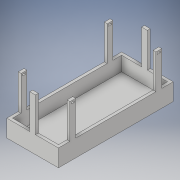
# Autodesk Inventor part: Part1
Saved by Autodesk Inventor 2017 (Build 210142000, 142)
## iProperties
Created: 2017-10-07
Part Number: Part1
Material: Generic
Document SubType Name: Modeling
Designer: User
Density: 1 g/cm^3
Appearance: Default
Author: User
Autodesk Inventor part; units mm, degrees
ref_plane "YZ Plane" through (0, 0, 0) normal (1, 0, 0) x (0, 1, 0)
ref_plane "XZ Plane" through (0, 0, 0) normal (0, 1, 0) x (-1, 0, 0)
ref_plane "XY Plane" through (0, 0, 0) normal (0, 0, 1) x (1, 0, 0)
sketch "Sketch1" plane through (0, 0, 0) normal (0, 1, 0) x (-1, 0, 0)
  line L0 (0, 0) -> (3.175, 0)
  line L1 (3.175, 0) -> (3.175, -3.175)
  line L2 (3.175, -3.175) -> (0, -3.175)
  line L3 (0, -3.175) -> (0, 0)
  line L4 (0, 0) -> (6.35, 0)
  line L5 (0, -6.35) -> (0, 0)
  line L6 (3.175, 0) -> (50.8, 0)
  line L7 (50.8, 0) -> (50.8, -3.175)
  line L8 (50.8, -3.175) -> (3.175, -3.175)
  line L9 (3.175, -3.175) -> (3.175, 0)
  line L10 (50.8, 0) -> (57.15, 0)
  line L11 (57.15, 0) -> (57.15, -6.35)
  line L12 (57.15, 0) -> (53.975, 0)
  line L13 (53.975, 0) -> (53.975, -3.175)
  line L14 (53.975, -3.175) -> (57.15, -3.175)
  line L15 (57.15, -3.175) -> (57.15, 0)
  line L16 (53.975, -120.65) -> (53.975, -123.825)
  line L17 (53.975, -123.825) -> (50.8, -123.825)
  line L18 (57.15, -120.65) -> (57.15, -127)
  line L19 (57.15, -127) -> (50.8, -127)
  line L20 (3.175, -120.65) -> (3.175, -123.825)
  line L21 (3.175, -123.825) -> (6.35, -123.825)
  line L22 (0, -120.65) -> (0, -127)
  line L23 (0, -127) -> (6.35, -127)
  line L24 (53.975, -127) -> (57.15, -127)
  line L25 (57.15, -127) -> (57.15, 0)
  line L26 (57.15, 0) -> (53.975, 0)
  line L27 (53.975, 0) -> (53.975, -127)
  line L28 (50.8, -3.175) -> (57.15, -3.175)
  line L29 (57.15, -3.175) -> (57.15, 0)
  line L30 (57.15, 0) -> (50.8, 0)
  line L31 (50.8, 0) -> (50.8, -3.175)
  line L32 (50.8, -127) -> (6.35, -127)
  line L33 (6.35, -127) -> (6.35, -123.825)
  line L34 (6.35, -123.825) -> (50.8, -123.825)
  line L35 (50.8, -123.825) -> (50.8, -127)
  line L36 (0, -120.65) -> (3.175, -120.65)
  line L37 (3.175, -120.65) -> (3.175, -6.35)
  line L38 (3.175, -6.35) -> (0, -6.35)
  line L39 (0, -6.35) -> (0, -120.65)
  line L40 (3.175, -6.35) -> (3.175, -3.175)
  line L41 (3.175, -3.175) -> (6.35, -3.175)
  line L42 (53.975, -123.825) -> (57.15, -123.825)
  line L43 (57.15, -123.825) -> (57.15, -120.65)
  line L44 (57.15, -120.65) -> (53.975, -120.65)
  line L45 (53.975, -120.65) -> (53.975, -123.825)
  line L46 (0, -127) -> (3.175, -127)
  line L47 (3.175, -127) -> (3.175, -123.825)
  line L48 (3.175, -123.825) -> (0, -123.825)
  line L49 (0, -123.825) -> (0, -127)
  line L50 (3.175, -3.175) -> (6.35, -3.175)
  line L51 (6.35, -3.175) -> (6.35, 0)
  line L52 (6.35, 0) -> (3.175, 0)
  line L53 (3.175, 0) -> (3.175, -3.175)
  line L54 (57.15, -3.175) -> (53.975, -3.175)
  line L55 (53.975, -3.175) -> (53.975, -6.35)
  line L56 (53.975, -6.35) -> (57.15, -6.35)
  line L57 (57.15, -6.35) -> (57.15, -3.175)
  line L58 (57.15, -6.35) -> (53.975, -6.35)
  line L59 (53.975, -6.35) -> (53.975, -120.65)
  line L60 (53.975, -120.65) -> (57.15, -120.65)
  line L61 (57.15, -120.65) -> (57.15, -6.35)
  line L62 (3.175, -3.175) -> (0, -3.175)
  line L63 (0, -3.175) -> (0, -6.35)
  line L64 (0, -6.35) -> (3.175, -6.35)
  line L65 (3.175, -6.35) -> (3.175, -3.175)
  line L66 (3.175, -123.825) -> (0, -123.825)
  line L67 (0, -123.825) -> (0, -120.65)
  line L68 (0, -120.65) -> (3.175, -120.65)
  line L69 (3.175, -120.65) -> (3.175, -123.825)
  line L70 (3.175, -123.825) -> (6.35, -123.825)
  line L71 (6.35, -123.825) -> (6.35, -127)
  line L72 (6.35, -127) -> (3.175, -127)
  line L73 (3.175, -127) -> (3.175, -123.825)
  line L74 (53.975, -123.825) -> (50.8, -123.825)
  line L75 (50.8, -123.825) -> (50.8, -127)
  line L76 (50.8, -127) -> (53.975, -127)
  line L77 (53.975, -127) -> (53.975, -123.825)
  line L78 (57.15, -120.65) -> (53.975, -120.65)
  line L79 (53.975, -120.65) -> (53.975, -123.825)
  line L80 (53.975, -123.825) -> (57.15, -123.825)
  line L81 (57.15, -123.825) -> (57.15, -120.65)
  dimension "d2" = 3.175
  dimension "d3" = 3.175
  dimension "d7" = 6.35
  dimension "d8" = 3.175
  dimension "d9" = 3.175
  dimension "d10" = 3.175
  dimension "d11" = 3.175
  dimension "d12" = 6.35
  dimension "d13" = 6.35
  dimension "d14" = 3.175
  dimension "d15" = 3.175
  dimension "d16" = 6.35
  dimension "d17" = 6.35
  dimension "d18" = 3.175
  constraints: 164 end point, 34 parallel, 19 horizontal, 18 perpendicular, 1 midpoint, 1 point on line
  measures "d2" distance of L1.end L2.end
  measures "d3" distance of L0.end L1.end
  measures "d7" distance of L10.end L11.end
  measures "d8" distance of L14.end L13.end
  measures "d9" distance of L13.end L12.end
  measures "d10" distance of L16.end L17.end
  measures "d11" distance of L16.start L16.end
  measures "d12" distance of L18.end L19.end
  measures "d13" distance of L18.start L18.end
  measures "d14" distance of L21.end L20.end
  measures "d15" distance of L20.end L20.start
  measures "d16" distance of L23.end L22.end
  measures "d17" distance of L22.end L22.start
  measures "d18" distance of L52.end L4.end
extrude "Extrusion1" add sketch "Sketch1" along normal blind 19.05 contours L0 L1 L2 L3 | L4 L51 L8 L1 | L2 L40 L38 L5 | L6 L7 L8 L51 | L38 L37 L36 L39 | L10 L13 L28 L7 | L36 L20 L48 L22 | L10 L11 L14 L13 | L48 L47 L23 L22 | L14 L11 L56 L27 | L21 L33 L23 L47 | L56 L25 L44 L27 | L34 L35 L32 L33 | L44 L18 L42 L16 | L17 L27 L19 L35 | L42 L18 L19 L27
sketch "Sketch2" plane through (0, 0, 0) normal (0, -1, 0) x (1, 0, 0)
  line L0 (-3.175, -3.175) -> (-53.975, -3.175) projected
  line L1 (-53.975, -123.825) -> (-3.175, -123.825)
  line L2 (-3.175, -123.825) -> (-3.175, -3.175)
  line L3 (-3.175, -3.175) -> (-53.975, -3.175)
  line L4 (-53.975, -3.175) -> (-53.975, -123.825)
  point P0 (0, 0)
  constraints: 8 end point, 2 parallel, 1 horizontal, 1 perpendicular
extrude "Extrusion2" add sketch "Sketch2" against normal blind 3.175
sketch "Sketch3" plane through (0, 19.05, 0) normal (0, 1, 0) x (1, 0, 0)
  line L0 (0, 127) -> (-57.15, 127) projected
  line L1 (-57.15, 0) -> (0, 0) projected
  line L2 (-3.175, 123.825) -> (-53.975, 123.825) projected
  line L3 (-57.15, 127) -> (-57.15, 0) projected
  line L4 (-3.175, 3.175) -> (-53.975, 3.175) projected
  line L5 (-3.175, 123.825) -> (-3.175, 3.175) projected
  line L6 (-53.975, 3.175) -> (-53.975, 123.825) projected
  line L7 (0, 0) -> (0, 127) projected
  line L8 (0, 114.3) -> (-3.175, 114.3)
  line L9 (-3.175, 114.3) -> (0, 114.3)
  line L10 (0, 114.3) -> (0, 107.95)
  line L11 (0, 107.95) -> (-3.175, 107.95)
  line L12 (-3.175, 107.95) -> (-3.175, 114.3)
  line L13 (0, 0) -> (0, 12.7)
  line L14 (0, 12.7) -> (-3.175, 12.7)
  line L15 (-3.175, 12.7) -> (0, 12.7)
  line L16 (0, 12.7) -> (0, 19.05)
  line L17 (0, 19.05) -> (-3.175, 19.05)
  line L18 (-3.175, 19.05) -> (-3.175, 12.7)
  line L19 (-53.975, 12.7) -> (-57.15, 12.7)
  line L20 (-57.15, 12.7) -> (-57.15, 19.05)
  line L21 (-57.15, 19.05) -> (-53.975, 19.05)
  line L22 (-53.975, 19.05) -> (-53.975, 12.7)
  line L23 (-53.975, 114.3) -> (-57.15, 114.3)
  line L24 (-57.15, 114.3) -> (-57.15, 107.95)
  line L25 (-57.15, 107.95) -> (-53.975, 107.95)
  line L26 (-53.975, 107.95) -> (-53.975, 114.3)
  line L27 (-31.75, 123.825) -> (-25.4, 123.825)
  line L28 (-25.4, 123.825) -> (-25.4, 127)
  line L29 (-25.4, 127) -> (-31.75, 127)
  line L30 (-31.75, 127) -> (-31.75, 123.825)
  line L31 (-31.75, 123.825) -> (-25.4, 127) construction
  line L32 (-25.4, 123.825) -> (-31.75, 127) construction
  line L33 (-31.75, 3.175) -> (-25.4, 3.175)
  line L34 (-25.4, 3.175) -> (-25.4, 0)
  line L35 (-25.4, 0) -> (-31.75, 0)
  line L36 (-31.75, 0) -> (-31.75, 3.175)
  line L37 (-31.75, 3.175) -> (-25.4, 0) construction
  line L38 (-25.4, 3.175) -> (-31.75, 0) construction
  point P0 (-28.575, 125.4125)
  point P1 (-28.575, 1.5875)
  dimension "d23" = 127
  dimension "d24" = 57.15
  dimension "d45" = 6.35
  dimension "d46" = 3.175
  dimension "d49" = 3.175
  dimension "d50" = 6.35
  dimension "d51" = 6.35
  dimension "d52" = 6.35
  dimension "d53" = 6.35
  dimension "d54" = 3.175
  dimension "d55" = 0
  dimension "d56" = 28.575
  dimension "d57" = 6.35
  dimension "d58" = 3.175
  dimension "d59" = 0
  dimension "d60" = 28.575
  dimension "d71" = 12.7
  dimension "d72" = 12.7
  dimension "d73" = 12.7
  dimension "d74" = 12.7
  constraints: 62 end point, 12 parallel, 6 horizontal, 6 perpendicular, 5 point on line, 4 midpoint
  measures "d23" distance between parallel lines of L0 L1
  measures "d24" distance of L0.start L0.end
  measures "d45" distance of L9.end L10.end
  measures "d46" distance of L14.end L13.end
  measures "d49" distance of L17.end L16.end
  measures "d50" distance of L16.end L15.end
  measures "d51" distance between parallel lines of L25 L23
  measures "d52" distance between parallel lines of L19 L21
  measures "d53" distance of L29.end L28.end
  measures "d54" distance of L28.end L27.end
  measures "d55" distance between parallel lines of L2 L27
  measures "d56" distance from line of L3 point (-28.575, 125.412)
  measures "d57" distance of L34.end L35.end
  measures "d58" distance of L33.end L34.end
  measures "d59" distance between parallel lines of L1 L35
  measures "d60" distance from line of L7 point (-28.575, 1.588)
  measures "d71" distance between parallel lines of L23 L0
  measures "d72" distance between parallel lines of L9 L0
  measures "d73" distance between parallel lines of L1 L14
  measures "d74" distance between parallel lines of L1 L19
extrude "Extrusion3" add sketch "Sketch3" along normal blind 38.1 contours L28 L2 L30 L0 | L7 L11 L5 L8 | L7 L14 L5 L17 | L23 L6 L25 L3 | L21 L6 L19 L3 | L1 L36 L4 L34
sketch "Sketch5" plane through (0, 0, 0) normal (1, 0, 0) x (0, 0, -1)
  line L0 (114.3, 19.05) -> (114.3, 57.15) projected
  line L1 (107.95, 19.05) -> (107.95, 57.15) projected
  line L2 (109.5375, 55.5625) -> (112.7125, 55.5625)
  line L3 (112.7125, 55.5625) -> (112.7125, 53.975)
  line L4 (112.7125, 53.975) -> (109.5375, 53.975)
  line L5 (109.5375, 53.975) -> (109.5375, 55.5625)
  line L6 (107.95, 57.15) -> (114.3, 57.15) projected
  line L7 (14.2875, 53.975) -> (17.4625, 53.975)
  line L8 (17.4625, 53.975) -> (17.4625, 55.5625)
  line L9 (17.4625, 55.5625) -> (14.2875, 55.5625)
  line L10 (14.2875, 55.5625) -> (14.2875, 53.975)
  line L11 (12.7, 19.05) -> (12.7, 57.15) projected
  line L12 (12.7, 57.15) -> (19.05, 57.15) projected
  point P0 (0, 0)
  dimension "d61" = 6.35
  dimension "d62" = 3.175
  dimension "d63" = 1.5875
  dimension "d64" = 1.5875
  dimension "d66" = 1.5875
  dimension "d67" = 3.175
  dimension "d68" = 1.5875
  dimension "d88" = 1.5875
  dimension "d89" = 1.5875
  constraints: 16 end point, 4 parallel, 2 horizontal, 2 perpendicular
  measures "d61" distance between parallel lines of L0 L1
  measures "d62" distance of L3.end L4.end
  measures "d63" distance of L2.end L3.end
  measures "d64" distance between parallel lines of L3 L0
  measures "d66" distance between parallel lines of L2 L6
  measures "d67" distance of L8.end L9.end
  measures "d68" distance between parallel lines of L11 L10
  measures "d88" distance between parallel lines of L12 L9
  measures "d89" distance between parallel lines of L7 L9
extrude "Extrusion4" cut sketch "Sketch5" against normal blind 25374.6
body "Solid1"
